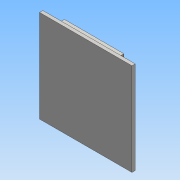
# Autodesk Inventor part: LCD5110
Saved by Autodesk Inventor 2016 (Build 200138000, 138)
## iProperties
Created: 2015-09-16
Part Number: LCD5110
Material: Generic
Document SubType Name: Modeling
Designer: Openlab
Density: 1 g/cm^3
Appearance: Default
Mass: 5.3735 g
Surface Area: 48.28 cm^2
Volume: 5.3735 cm^3
Author: Openlab
Autodesk Inventor part; units mm, degrees
ref_plane "YZ Plane" through (0, 0, 0) normal (1, 0, 0) x (0, 1, 0)
ref_plane "XZ Plane" through (0, 0, 0) normal (0, 1, 0) x (-1, 0, 0)
ref_plane "XY Plane" through (0, 0, 0) normal (0, 0, 1) x (1, 0, 0)
sketch "Sketch1" plane through (0, 0, 0) normal (0, 1, 0) x (-1, 0, 0)
  line L0 (-22.5, 22.5) -> (22.5, 22.5)
  line L1 (22.5, 22.5) -> (22.5, -22.5)
  line L2 (22.5, -22.5) -> (-22.5, -22.5)
  line L3 (-22.5, -22.5) -> (-22.5, 22.5)
  line L4 (-22.5, 22.5) -> (22.5, -22.5) construction
  line L5 (22.5, 22.5) -> (-22.5, -22.5) construction
  line L6 (-14.5, 21.5) -> (14.5, 21.5)
  line L7 (14.5, 21.5) -> (14.5, -21.5)
  line L8 (14.5, -21.5) -> (-14.5, -21.5)
  line L9 (-14.5, -21.5) -> (-14.5, 21.5)
  line L10 (-14.5, 21.5) -> (14.5, -21.5) construction
  line L11 (14.5, 21.5) -> (-14.5, -21.5) construction
  point P0 (0, 0)
  dimension "d0" = 45
  dimension "d1" = 45
  dimension "d2" = 29
  dimension "d3" = 43
  constraints: 24 end point, 4 midpoint, 4 parallel, 2 horizontal, 2 perpendicular
  measures "d0" distance of L1.end L2.end
  measures "d1" distance of L0.end L1.end
  measures "d2" distance of L7.end L8.end
  measures "d3" distance of L6.end L7.end
extrude "Extrusion1" add sketch "Sketch1" against normal blind 1.6 contours L0 L1 L2 L3 | L6 L7 L8 L9
extrude "Extrusion2" add sketch "Sketch1" along normal blind 2.5 contours L6 L7 L8 L9
sketch "Sketch2" plane through (0, 2.5, 0) normal (0, 1, 0) x (1, 0, 0)
  line L0 (12, -20.5) -> (-12, -20.5)
  line L1 (-12, -20.5) -> (-12, 20.5)
  line L2 (-12, 20.5) -> (12, 20.5)
  line L3 (12, 20.5) -> (12, -20.5)
  line L4 (12, -20.5) -> (-12, 20.5) construction
  line L5 (-12, -20.5) -> (12, 20.5) construction
  point P0 (0, 0)
  dimension "d8" = 24
  dimension "d9" = 41
  constraints: 12 end point, 2 midpoint, 2 parallel, 1 horizontal, 1 perpendicular
  measures "d8" distance of L1.end L2.end
  measures "d9" distance of L0.end L1.end
extrude "Extrusion3" cut sketch "Sketch2" against normal blind 1
body "Solid1"
